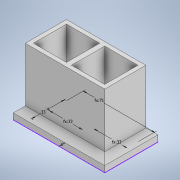
# Autodesk Inventor part: double
Saved by Autodesk Inventor 2022 (Build 260153000, 153)
## iProperties
Created: 2021-10-08
Part Number: double
Material: Generic
Document SubType Name: Modeling
Designer: dangl
Density: 1 g/cm^3
Appearance: Default
Author: dangl
Autodesk Inventor part; units mm, degrees
ref_plane "YZ Plane" through (0, 0, 0) normal (1, 0, 0) x (0, 1, 0)
ref_plane "XZ Plane" through (0, 0, 0) normal (0, 1, 0) x (-1, 0, 0)
ref_plane "XY Plane" through (0, 0, 0) normal (0, 0, 1) x (1, 0, 0)
sketch "Sketch1" plane through (0, 0, 0) normal (0, 1, 0) x (-1, 0, 0)
  line L0 (0, 0) -> (33, 0)
  line L1 (71, 0) -> (71, -33)
  line L2 (71, -33) -> (38, -33)
  line L3 (0, -33) -> (0, 0)
  line L4 (0, -33) -> (0, 0)
  line L5 (75, -37) -> (75, 4)
  line L6 (75, 4) -> (-4, 4)
  line L7 (-4, 4) -> (-4, -37)
  line L8 (-4, -37) -> (75, -37)
  line L9 (-10, 10) -> (81, 10)
  line L10 (81, 10) -> (81, -43)
  line L11 (81, -43) -> (-10, -43)
  line L12 (-10, -43) -> (-10, 10)
  line L13 (38, -33) -> (38, 0)
  line L14 (33, -33) -> (33, 0)
  line L15 (38, -33) -> (33, -33)
  line L16 (33, -33) -> (0, -33)
  line L17 (38, 0) -> (71, 0)
  line L18 (33, 0) -> (38, 0)
  point P0 (0, -33)
  point P1 (0, -37)
  point P2 (0, 4)
  dimension "d0" = 33
  dimension "d1" = 71
  dimension "d5" = 4
  dimension "d10" = 6
  dimension "d19" = 33
  dimension "d20" = 33
  constraints: 38 end point, 14 parallel, 11 perpendicular, 3 horizontal, 2 point on line, 3 other
  measures "d0" distance of L1.start L1.end
  measures "d1" distance of L3.start L1.end
  measures "d5" distance between parallel lines of L1 L5
  measures "d10" distance between parallel lines of L6 L9
  measures "d19" distance between parallel lines of L1 L13
  measures "d20" distance between parallel lines of L3 L14
extrude "Extrusion1" add sketch "Sketch1" along normal blind 6 contours L0 L14 L16 L3 | L18 L13 L15 L14 | L17 L1 L2 L13 | L8 L7 L6 L5 | L9 L10 L11 L12
extrude "Extrusion4" add sketch "Sketch1" along normal blind 66 contours L18 L13 L15 L14 | L8 L7 L6 L5
chamfer "Chamfer3" distance 6 angle 45 4 edges at (-75, 6, -16.5) (-35.5, 6, 4) (4, 6, -16.5) (-35.5, 6, -37)
equation "\"d19\" = d0"
equation "\"d20\" = d19"
body "Solid1"
